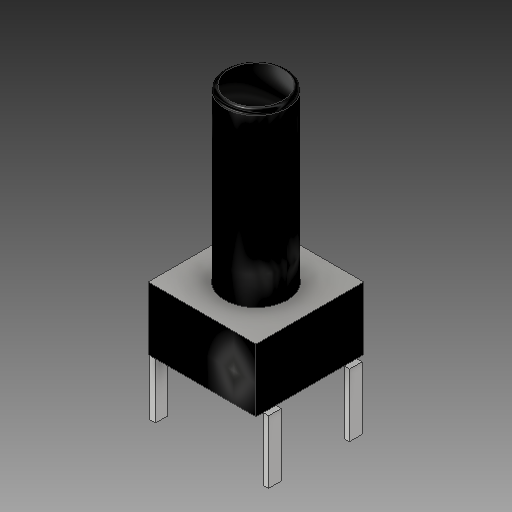
# Autodesk Inventor part: Touch Button High
Saved by Autodesk Inventor 2019 (Build 230136000, 136)
## iProperties
Created: 2018-06-11
Part Number: Touch Button High
Material: Générique
Document SubType Name: Modeling
Designer: dimercur
Density: 1 g/cm^3
Appearance: Par défaut
Author: dimercur
Autodesk Inventor part; units mm, degrees
ref_plane "YZ Plane" through (0, 0, 0) normal (1, 0, 0) x (0, 1, 0)
ref_plane "XZ Plane" through (0, 0, 0) normal (0, 1, 0) x (-1, 0, 0)
ref_plane "XY Plane" through (0, 0, 0) normal (0, 0, 1) x (1, 0, 0)
sketch "Esquisse1" plane through (0, 0, 0) normal (0, 1, 0) x (-1, 0, 0)
  line L0 (3, -3) -> (-3, -3)
  line L1 (-3, -3) -> (-3, 3)
  line L2 (-3, 3) -> (3, 3)
  line L3 (3, 3) -> (3, -3)
  point P0 (0, 0)
  dimension "d0" = 6
  dimension "d1" = 6
  dimension "d2" = 3
  dimension "d3" = 3
  constraints: 8 end point, 2 parallel, 1 horizontal, 1 perpendicular
  measures "d0" distance of L0.start L0.end
  measures "d1" distance of L2.end L0.start
  measures "d2" horizontal distance of point (0, 0) L0.start
  measures "d3" horizontal distance of point (0, 0) L0.start
extrude "Extrusion1" add sketch "Esquisse1" along normal blind 3.5
sketch "Esquisse2" plane through (0, 3.5, 0) normal (0, 1, 0) x (1, 0, 0)
  circle A0 centre (0, 0) radius 1.75
  dimension "d6" = 3.5
  constraints: 1 centre point, 1 coincident
  measures "d6" diameter of A0
extrude "Extrusion2" add sketch "Esquisse2" along normal blind 9.5
fillet "Congé1" radius 0.25 1 edges at (-1.75, 13, 0)
sketch "Esquisse3" plane through (0, 0, 0) normal (0, -1, 0) x (1, 0, 0)
  line L0 (3, 3) -> (3, -3) projected
  line L1 (3, 2.6) -> (3.3, 2.6)
  line L2 (3.3, 2.6) -> (3.3, 1.9)
  line L3 (3.3, 1.9) -> (3, 1.9)
  line L4 (3, 1.9) -> (3, 2.6)
  line L5 (3, -1.9) -> (3.3, -1.9)
  line L6 (3.3, -1.9) -> (3.3, -2.6)
  line L7 (3.3, -2.6) -> (3, -2.6)
  line L8 (3, -2.6) -> (3, -1.9)
  line L9 (-3, -3) -> (-3, 3) projected
  line L10 (-3, 2.6) -> (-3.3, 2.6)
  line L11 (-3.3, 2.6) -> (-3.3, 1.9)
  line L12 (-3.3, 1.9) -> (-3, 1.9)
  line L13 (-3, 1.9) -> (-3, 2.6)
  line L14 (-3, -1.9) -> (-3.3, -1.9)
  line L15 (-3.3, -1.9) -> (-3.3, -2.6)
  line L16 (-3.3, -2.6) -> (-3, -2.6)
  line L17 (-3, -2.6) -> (-3, -1.9)
  point P0 (0, 0)
  dimension "d11" = 0.7
  dimension "d12" = 0.3
  dimension "d13" = 0.7
  dimension "d14" = 0.3
  dimension "d15" = 3.8
  dimension "d16" = 6
  dimension "d17" = 0.4
  dimension "d18" = 0.7
  dimension "d19" = 0.7
  dimension "d20" = 3.8
  dimension "d21" = 0.3
  dimension "d22" = 0.3
  dimension "d23" = 0.4
  constraints: 32 end point, 8 parallel, 4 horizontal, 4 perpendicular, 4 point on line
  measures "d11" distance of L1.end L2.end
  measures "d12" distance of L1.start L1.end
  measures "d13" distance of L5.end L6.end
  measures "d14" distance of L5.start L5.end
  measures "d15" distance between parallel lines of L3 L5
  measures "d16" distance of L0.start L0.end
  measures "d17" distance from line of L0.start L1
  measures "d18" distance of L10.end L11.end
  measures "d19" distance of L14.end L15.end
  measures "d20" distance between parallel lines of L14 L12
  measures "d21" distance of L10.start L10.end
  measures "d22" distance of L15.end L16.end
  measures "d23" distance from line of L10 L9.end
extrude "Extrusion3" add sketch "Esquisse3" along normal blind 3.5
equation "\"d1\" = d0"
equation "\"d2\" = 0.5 * d0"
equation "\"d3\" = 0.5 * d1"
equation "\"d13\" = d11"
equation "\"d14\" = d12"
equation "\"d17\" = -0.5 * d15 + 0.5 * d16 - d11"
equation "\"d18\" = d11"
equation "\"d19\" = d11"
equation "\"d20\" = d15"
equation "\"d21\" = d12"
equation "\"d22\" = d21"
equation "\"d23\" = d17"
